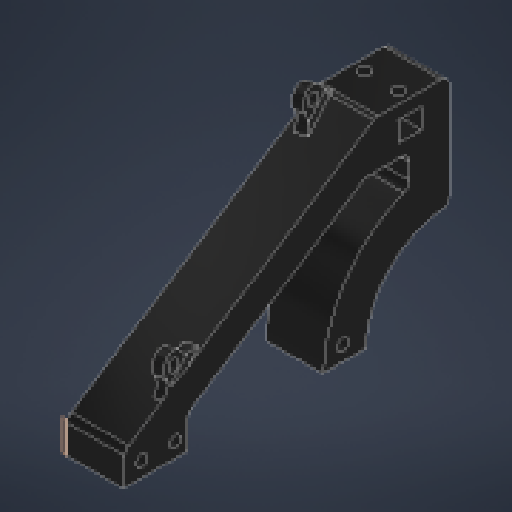
# Autodesk Inventor part: Funnel
Saved by Autodesk Inventor 2026.1 (Build 301233000, 233)
## iProperties
Created: 2025-09-08
Part Number: Funnel
Material: Plastic, Opaque Black
Document SubType Name: Modeling
Designer: Teddy
Density: 0.952 g/cm^3
Appearance: Smooth - Black
Author: Teddy
Autodesk Inventor part; units mm, degrees
ref_plane "YZ Plane" through (0, 0, 0) normal (1, 0, 0) x (0, 1, 0)
ref_plane "XZ Plane" through (0, 0, 0) normal (0, 1, 0) x (-1, 0, 0)
ref_plane "Work Plane1" through (-22.225, 0, 0) normal (0, 0, 1) x (1, 0, 0)
sketch "Sketch1" plane through (-22.225, 0, 0) normal (0, 0, 1) x (1, 0, 0)
  line L0 (0, 0) -> (0, 10.8902) projected
  arc A0 (0, 0) -> (0.7937, -0.7938) centre (0.7937, 0) ccw projected
  line L1 (8.8011, -0.7938) -> (0.7937, -0.7938) projected
  arc A1 (21.4312, -0.7938) -> (22.225, 0) centre (21.4313, 0) ccw projected
  line L2 (22.225, 0) -> (22.225, 10.8902) projected
  line L3 (21.4312, -0.7938) -> (8.8011, -0.7938)
  line L4 (21.4312, 73.8188) -> (13.4239, 73.8188) projected
  line L5 (0.254, 10.8902) -> (0.254, 0)
  arc A2 (0.254, 0) -> (0.7938, -0.5398) centre (0.7937, 0) ccw
  line L6 (0.7938, -0.5398) -> (8.8011, -0.5398)
  line L7 (8.8011, -0.5398) -> (21.4313, -0.5398)
  arc A3 (21.4313, -0.5398) -> (21.971, 0) centre (21.4313, 0) ccw
  line L8 (21.971, 0) -> (21.971, 10.8902)
  line L9 (0.254, 10.8902) -> (0.254, 73.8188)
  line L10 (0.254, 73.8188) -> (21.4312, 73.8188)
  line L11 (21.971, 10.8902) -> (21.971, 73.8188)
  line L12 (21.971, 73.8188) -> (21.4312, 73.8188)
  dimension "d0" = 0.254
  constraints: 18 end point, 4 point on circle, 2 centre point, 2 perpendicular, 2 point on line, 1 collinear, 1 horizontal, 1 horizontal alignment, 5 other
  measures "d0" distance between parallel lines of L1 L6
ref_plane "Work Plane2" through (-6.5659, 73.8187, -122.9614) normal (0, 0, 1) x (1, 0, 0)
extrude "Extrusion1" add sketch "Sketch1" against normal up to surface (122.9614 mm away)
sketch "Sketch2" plane through (-21.971, 0, 0) normal (-1, 0, 0) x (0, 0, 1)
  circle A0 centre (-19.05, 5.5562) radius 2.1844 projected
  line L0 (0, 73.8188) -> (0, 0) projected
  line L1 (0, 12.1602) -> (-95.0214, 73.8188)
  line L2 (0, 73.8188) -> (-122.9614, 73.8188) projected
  line L3 (0, -0.5398) -> (-122.9614, -0.5398) projected
  line L4 (0, 12.1602) -> (0, 73.8188)
  line L5 (-95.0214, 73.8188) -> (0, 73.8188)
  circle A1 centre (-122.9614, -0.5398) radius 31.75
  line L6 (0, -0.5398) -> (-122.9614, -0.5398) projected
  line L7 (-23.7228, -0.5398) -> (-23.7228, 12.4143)
  line L8 (-23.7228, 12.4143) -> (-90.9521, 56.0387)
  line L9 (-90.9521, 56.0387) -> (-107.7214, 56.0387)
  line L10 (-107.7214, 56.0387) -> (-107.7214, 27.3135)
  circle A2 centre (-122.9614, -0.5398) radius 47.625
  line L11 (-91.2114, -0.5398) -> (-75.3364, -0.5398)
  line L12 (-122.9614, 0) -> (-122.9614, 73.8188) projected
  line L13 (-122.9614, 31.2102) -> (-122.9614, 73.8188)
  line L14 (-122.9614, 73.8188) -> (-95.0214, 73.8188)
  circle A3 centre (-82.55, 5.5563) radius 2.1844 projected
  circle A4 centre (-6.35, 5.5562) radius 2.1844 projected
  point P0 (-107.7214, 44.581)
  point P1 (-75.3364, -0.5398)
  dimension "d6" = 95.25
  dimension "d3" = 27.94
  dimension "d4" = 12.7
  dimension "d5" = 63.5
  dimension "d7" = 12.7
  dimension "d8" = 17.78
  dimension "d9" = 15.24
  constraints: 20 end point, 5 perpendicular, 5 point on line, 3 point on circle, 2 coincident, 2 collinear, 1 centre point, 3 other
  measures "d3" distance of L2.end L1.end
  measures "d4" distance from line of L3 L1.start
  measures "d5" diameter of A1
  measures "d7" distance between parallel lines of L1 L8
  measures "d8" distance between parallel lines of L14 L9
  measures "d9" distance between parallel lines of L12 L10
extrude "Extrusion2" cut sketch "Sketch2" against normal blind 25.4 contours A0 | L0 L1 L2 | L3 A2 L10 L9 L8 L7 | A1 | A3 | A4
fillet "Fillet1" radius 3.175 8 edges at (-11.1125, 31.2102, -122.9614) (-11.1125, 56.0387, -107.7214) (-11.1125, 56.0387, -90.9521) (-11.1125, 44.581, -107.7214) (-11.1125, 12.4143, -23.7228) (-11.1125, 12.1602, 0) (-11.1125, 73.8187, -95.0214) (-11.1125, 73.8187, -122.9614)
sketch "Sketch3" plane through (-21.971, 0, -23.7228) normal (-1, 0, 0) x (0, 0, 1)
  line L0 (-79.7696, 68.7388) -> (-88.5326, 68.7388)
  line L1 (-88.5326, 68.7388) -> (-88.5326, 61.1188)
  line L2 (-88.5326, 61.1188) -> (-79.7696, 61.1188)
  line L3 (-79.7696, 61.1188) -> (-79.7696, 68.7388)
  line L4 (-81.9158, 73.8188) -> (-81.9158, 75.4063) projected
  line L5 (-86.5386, 73.8188) -> (-86.5386, 75.4063) projected
  line L6 (-72.2385, 73.8188) -> (-96.0636, 73.8188) projected
  line L7 (-84.1511, 73.8188) -> (-84.1511, 59.9526) construction
  point P0 (23.7228, 0)
  dimension "d13" = 7.62
  dimension "d14" = 8.763
  dimension "d15" = 5.08
  constraints: 10 end point, 2 parallel, 2 perpendicular, 1 horizontal, 1 midpoint, 1 other
  measures "d13" distance of L2.end L0.start
  measures "d14" distance between parallel lines of L1 L3
  measures "d15" distance between parallel lines of L6 L0
extrude "Extrusion3" cut sketch "Sketch3" against normal blind 25.4
sketch "Sketch4" plane through (-21.971, 73.8187, -119.7864) normal (0, 1, 0) x (1, 0, 0)
  circle A0 centre (4.5085, -11.8364) radius 2.1844 projected
  circle A1 centre (17.2085, -11.8364) radius 2.1844 projected
  point P0 (21.971, -119.7864)
extrude "Extrusion4" cut sketch "Sketch4" against normal up to surface (5.08 mm away)
ref_plane "Work Plane3" through (-0.254, 0, 0) normal (-0.9528685, 0, 0.3033835) x (0, 1, 0)
sketch "Sketch7" plane through (-0.254, 0, 0) normal (-0.9528685, 0, 0.3033835) x (0, 1, 0)
  circle A0 centre (29.2784, 19.3161) radius 6.985
  circle A1 centre (57.872, 61.3047) radius 6.985
  line L0 (13.099, 7.9671) -> (73.3072, 96.3802) projected
  line L1 (73.3072, 89.7917) -> (13.099, 1.3786) projected
  circle A2 centre (29.2784, 19.3161) radius 2.286
  circle A3 centre (57.872, 61.3047) radius 2.286
  line L2 (35.9904, 21.2498) -> (31.8741, 35.5376)
  line L3 (28.549, 12.3693) -> (16.9278, 13.5895)
  line L4 (16.9278, 13.5895) -> (31.8741, 35.5376)
  ellipse E0 centre (10.4356, 9.6139) end of major axis (7.2606, 9.6139) minor radius 3.0254 (10.4356, 6.5886) -> (13.099, 7.9671) ccw projected
  line L5 (52.0986, 65.2364) -> (54.6063, 68.9188)
  line L6 (54.6063, 68.9188) -> (55.4048, 70.0914)
  line L7 (55.4048, 70.0914) -> (60.755, 67.667)
  line L8 (57.872, 54.3197) -> (45.6235, 55.7279)
  line L9 (55.4048, 70.0914) -> (45.6235, 55.7279)
  point P0 (0, -0.0771)
  point P1 (11.9377, 6.9486)
  point P2 (61.863, 74.9638)
  point P3 (63.1249, 76.867)
  point P4 (54.6063, 68.9188)
  point P5 (16.9278, 13.5895)
  point P6 (33.9323, 28.3937)
  point P7 (22.7384, 12.9794)
  point P8 (56.2869, 54.502)
  dimension "d33" = 13.97
  dimension "d34" = 13.97
  dimension "d35" = 4.572
  dimension "d36" = 4.572
  dimension "d37" = 17.3406
  dimension "d40" = 19.05
  dimension "d41" = 50.8
  constraints: 16 end point, 6 tangent, 5 point on circle, 4 centre point, 3 point on line, 2 coincident, 2 collinear, 2 midpoint, 1 parallel, 2 other
  measures "d33" diameter of A0
  measures "d34" diameter of A1
  measures "d35" diameter of A2
  measures "d36" diameter of A3
  measures "d37" horizontal distance of point (11.938, 6.949) A0.centre
  measures "d40" distance of point (33.932, 28.394) point (22.738, 12.979)
  measures "d41" distance of A3.centre A2.centre
extrude "Extrusion7" add sketch "Sketch7" against normal up to surface contours A0 L1 | A0 L1 L2 | L3 L1 A0 | L1 A0 | A0 L0 L2 L1 | L1 L3 L0 A0 | L8 L0 A1 L1 | L1 A1 L8 | L1 A1 L8 | A1 L1 | L8 A1 | L0 L7 L1 A1 | L1 L7 A1 surface through (-0.254, 73.8188, 0) normal (1, 0, 0)
body "Solid1"
